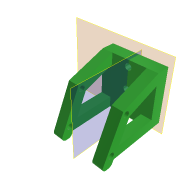
# Autodesk Inventor part: Gripper_linear_finger
Saved by Autodesk Inventor 2022 (Build 260153000, 153)
## iProperties
Created: 2023-01-05
Part Number: Gripper_linear_finger
Material: Generisch
Document SubType Name: Modeling
Designer: diederichbenedict
Density: 1 g/cm^3
Appearance: Glatt - Waldgrün
Author: diederichbenedict
Autodesk Inventor part; units mm, degrees
ref_plane "YZ Plane" through (0, 0, 0) normal (1, 0, 0) x (0, 1, 0)
ref_plane "XZ Plane" through (0, 0, 0) normal (0, 1, 0) x (-1, 0, 0)
ref_plane "XY Plane" through (0, 0, 0) normal (0, 0, 1) x (1, 0, 0)
ref_plane "Arbeitsebene1" through (0, 0, 0) normal (0, 0, 1) x (1, 0, 0)
sketch "Skizze1" plane through (0, 0, 0) normal (0, 0, 1) x (1, 0, 0)
  circle A0 centre (19.6, 0) radius 1.5 projected
  circle A1 centre (9.6, 0) radius 1.5 projected
  circle A2 centre (-0.4, 0) radius 1.5 projected
  circle A3 centre (9.6, -10) radius 1.5 projected
  circle A4 centre (9.6, 10) radius 1.5 projected
  arc A5 (22.5, -8.5328) -> (22.5, -11.4672) centre (19.6, -10) ccw projected
  arc A6 (22.5, 11.4672) -> (17.6036, 7.4354) centre (19.6, 10) ccw projected
  line L0 (-3.3, 16.2) -> (-22.5, 16.2) projected
  line L1 (-22.5, 16.2) -> (-22.5, -16.2) projected
  line L2 (-22.5, -16.2) -> (22.5, -16.2) projected
  line L3 (22.5, -16.2) -> (22.5, -11.4672) projected
  circle A7 centre (-0.4, -10) radius 3.25 projected
  line L4 (-3.4, -13) -> (22.6, -13)
  line L5 (22.6, -13) -> (22.6, 13)
  line L6 (22.6, 13) -> (-3.4, 13)
  line L7 (-3.4, 13) -> (-3.4, -13)
  line L8 (-3.4, -13) -> (22.6, 13) construction
  line L9 (22.6, -13) -> (-3.4, 13) construction
  arc A8 (1.5964, 7.4354) -> (-2.3964, 7.4354) centre (-0.4, 10) ccw projected
  arc A9 (-2.3964, 7.4354) -> (1.5964, 7.4354) centre (-0.4, 4.8709) ccw projected
  arc A10 (-3.3, 23.4037) -> (-3.3, 26.3381) centre (-0.4, 24.8709) ccw projected
  line L10 (-3.3, 23.4037) -> (-3.3, 16.2) projected
  line L11 (22.5, -8.5328) -> (22.5, 3.4037) projected
  arc A11 (17.6036, 7.4354) -> (22.5, 3.4037) centre (19.6, 4.8709) ccw projected
  line L12 (22.5, 11.4672) -> (22.5, 23.4037) projected
  arc A12 (22.5, 26.3381) -> (22.5, 23.4037) centre (19.6, 24.8709) ccw projected
  line L13 (22.5, 26.3381) -> (22.5, 28.2) projected
  line L14 (22.5, 28.2) -> (-3.3, 28.2) projected
  line L15 (-3.3, 28.2) -> (-3.3, 26.3381) projected
  point P0 (0, 0)
  point P1 (22.5, 16.2)
  dimension "d0" = 26
  dimension "d1" = 26
  constraints: 12 end point, 2 midpoint, 2 parallel, 1 horizontal, 1 perpendicular
  measures "d0" distance of L6.end L5.end
  measures "d1" distance of L5.end L4.end
extrude "Extrusion1" add sketch "Skizze1" along normal blind 6 contours L11 A11 A6 L6 L12 L5 L4 L3 A5 | A5 L4 A7 L7 A9 A8 L6 A6 A11 L11 | A5 L3 L4 | L4 A7 L7 | L4 L7 A7 | L6 L12 A6 | A8 A9 L7 L6 | A8 L7 L6 | L7 A8 A9
sketch "Skizze2" plane through (-3.4, -13, 0) normal (-1, 0, 0) x (0, 0, 1)
  line L0 (0, 26) -> (0, 0) projected
  line L1 (0, 0) -> (6, 0) projected
  line L2 (6, 26) -> (6, 0) projected
  line L3 (0, 26) -> (6, 26) projected
  line L4 (6, 26) -> (23.9972, 19.4291)
  line L5 (23.9972, 19.4291) -> (32.8468, 0)
  line L6 (32.8468, 0) -> (27.3526, 0)
  line L7 (6, 24.5) -> (6, 20.6772)
  line L8 (27.3526, 0) -> (6, 0)
  line L9 (6, 20.6772) -> (20.3151, 15.4507)
  line L10 (20.3151, 15.4507) -> (25.0752, 5)
  line L11 (25.0752, 5) -> (6, 5)
  line L12 (32.8468, 0) -> (32.7967, 0.1099)
  line L13 (30.9766, -2.7191) -> (29.8778, -2.7191)
  line L14 (28.0577, -1.5481) -> (27.3526, 0)
  arc A0 (30.9766, -2.7191) -> (32.7967, 0.1099) centre (30.9766, -0.7191) ccw
  arc A1 (28.0577, -1.5481) -> (29.8778, -2.7191) centre (29.8778, -0.7191) ccw
  circle A2 centre (28.7957, 2.7835) radius 1.4
  circle A3 centre (22.3001, 17.2899) radius 1.4
  point P0 (0, 13)
  point P1 (32.8429, 0)
  point P2 (32.7967, 0.1099)
  dimension "d4" = 5
  dimension "d6" = 5
  dimension "d7" = 5
  dimension "d8" = 0
  dimension "d9" = 2
  dimension "d12" = 2.8
  dimension "d13" = 2.8
  constraints: 22 end point, 4 centre point, 4 point on circle, 4 tangent, 3 collinear, 3 parallel, 2 horizontal, 1 equal radius, 1 perpendicular, 1 point on line
  measures "d4" distance between parallel lines of L10 L5
  measures "d6" distance between parallel lines of L4 L9
  measures "d7" distance between parallel lines of L8 L11
  measures "d8" distance between parallel lines of L10 L14
  measures "d9" radius of A0
  measures "d12" diameter of A2
  measures "d13" diameter of A3
extrude "Extrusion2" add sketch "Skizze2" against normal blind 5 contours L3 L2 L1 L0 | L4 L5 A0 L6 L8 L2 L11 L10 L9 | L6 A0 L13 A1 L14
ref_plane "Arbeitsebene2" through (9.6, -13, 0) normal (-1, 0, 0) x (0, 0, 1)
mirror "Spiegeln1" about plane through (9.6, -13, 0) normal (-1, 0, 0) of "Extrusion2"
